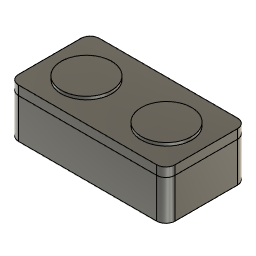
HCSR04-cover (Autodesk Fusion 360 design; units mm, degrees)
Autodesk Fusion 360 part; units mm, degrees
sketch "HCSR04-mock" plane through (0, 0, 0) normal (0, 0, 1) x (1, 0, 0)
  line L0 (0, 0) -> (45.3, 0)
  line L1 (45.3, 0) -> (45.3, 20.5)
  line L2 (45.3, 20.5) -> (0, 20.5)
  line L3 (0, 20.5) -> (0, 0)
  line L4 (22.65, 20.5) -> (22.65, 0) construction
  line L5 (17.525, 3.4) -> (27.775, 3.4)
  line L6 (27.775, 3.4) -> (27.775, 0.4)
  line L7 (27.775, 0.4) -> (17.525, 0.4)
  line L8 (17.525, 0.4) -> (17.525, 3.4)
  line L9 (17.275, 19.75) -> (28.025, 19.75)
  line L10 (28.025, 19.75) -> (28.025, 15.41)
  line L11 (28.025, 15.41) -> (17.275, 15.41)
  line L12 (17.275, 15.41) -> (17.275, 19.75)
  circle A0 centre (9.525, 9.75) radius 8.25
  line L13 (9.525, 9.75) -> (17.775, 9.75) construction
  circle A1 centre (35.775, 9.75) radius 8.25
  line L14 (35.775, 9.75) -> (27.525, 9.75) construction
  line L15 (9.525, 18) -> (9.525, 9.75) construction
  line L16 (35.775, 9.75) -> (35.775, 18)
  line L17 (17.775, 9.75) -> (27.525, 9.75) construction
  line L18 (27.05, 11.795) -> (18.25, 11.795)
  line L19 (18.25, 11.795) -> (18.25, 7.705)
  line L20 (18.25, 7.705) -> (27.05, 7.705)
  line L21 (27.05, 7.705) -> (27.05, 11.795)
  line L22 (27.05, 11.795) -> (18.25, 7.705) construction
  line L23 (18.25, 11.795) -> (27.05, 7.705) construction
  point P0 (22.65, 3.4)
  point P1 (22.65, 19.75)
  point P2 (17.775, 9.75)
  point P3 (27.525, 9.75)
  point P4 (9.525, 18)
  point P5 (35.775, 18)
  point P6 (22.65, 9.75)
  point P7 (22.65, 9.75)
  dimension "d40" = 45.3
  dimension "d41" = 20.5
  dimension "d44" = 10.25
  dimension "d45" = 3
  dimension "d46" = 0.4
  dimension "d47" = 10.75
  dimension "d48" = 4.34
  dimension "d49" = 0.75
  dimension "d50" = 16.5
  dimension "d51" = 16.5
  dimension "d52" = 2.5
  dimension "d53" = 2.5
  dimension "d55" = 9.75
  dimension "d69" = 8.8
  dimension "d70" = 4.09
  constraint horizontal L0
  constraint vertical L1
  constraint horizontal L2
  constraint vertical L3
  constraint coincident L0.start L3.end
  constraint midpoint L2 L4.start
  constraint midpoint L0 L4.end
  constraint horizontal L5
  constraint vertical L6
  constraint horizontal L7
  constraint vertical L8
  constraint midpoint L5 P0
  constraint coincident L4 P0
  constraint horizontal L9
  constraint vertical L10
  constraint horizontal L11
  constraint vertical L12
  constraint midpoint L9 P1
  constraint coincident L4 P1
  constraint coincident A0.centre L13.start
  constraint coincident A0 P2
  constraint horizontal L13
  constraint coincident A1.centre L14.start
  constraint coincident A1 P3
  constraint parallel L11 L14
  constraint coincident P2 L13.end
  constraint coincident P3 L14.end
  constraint coincident A0 P4
  constraint coincident P4 L15.start
  constraint perpendicular L13 L15
  constraint coincident A1 P5
  constraint perpendicular L14 L16
  constraint coincident P5 L16.end
  constraint midpoint L17 P7
  constraint coincident L4 P7
  constraint horizontal L18
  constraint perpendicular L18 L19
  constraint parallel L18 L20
  constraint parallel L19 L21
  constraint coincident L22 P7
  constraint coincident L23 P7
  constraint coincident P7 P6
  measures "d40" distance of L0.start L0.end
  measures "d41" distance of L0.start L2.end
  measures "d44" distance of L5.start L5.end
  measures "d45" distance of L5.start L7.end
  measures "d46" distance of L0 L7
  measures "d47" distance of L9.start L9.end
  measures "d48" distance of L9.start L11.end
  measures "d49" distance of L2 L9
  measures "d50" diameter of A0
  measures "d51" diameter of A1
  measures "d52" distance of L2 P4
  measures "d53" distance of L2 P5
  measures "d55" distance of P2 P3
  measures "d69" distance of L19.end L20.end
  measures "d70" distance of L18.end L19.end
extrude "Extrude9" add sketch "HCSR04-mock" along normal blind 1.2 contours L0 L1 L2 L3 | L5 L6 L7 L8 | L9 L10 L11 L12 | A0 | A1 | L18 L19 L20 L21 makes body 1
extrude "Extrude10" add sketch "HCSR04-mock" along normal blind 12 from surface at 1.2 contours A0 | A1 bodies 1
extrude "Extrude11" add sketch "HCSR04-mock" along normal blind 3.6 from surface at 1.2 contours L9 L10 L11 L12 bodies 1
extrude "Extrude12" add sketch "HCSR04-mock" along normal blind 1.78 from surface at 1.2 contours L5 L6 L7 L8 bodies 1
extrude "Extrude13" add sketch "HCSR04-mock" against normal blind 1.8 contours L5 L6 L7 L8 bodies 1
extrude "Extrude14" add sketch "HCSR04-mock" against normal blind 1.75 contours L18 L19 L20 L21 bodies 1
sketch "Sketch5" plane through (0, 0, 1.2) normal (0, 0, 1) x (-1, 0, 0)
  line L0 (-17.525, -3.4) -> (-27.775, -3.4)
  line L1 (-27.775, -3.4) -> (-27.775, -0.4)
  line L2 (-27.775, -0.4) -> (-17.525, -0.4)
  line L3 (-17.525, -0.4) -> (-17.525, -3.4)
  line L4 (-17.275, -19.75) -> (-28.025, -19.75)
  line L5 (-28.025, -19.75) -> (-28.025, -15.41)
  line L6 (-28.025, -15.41) -> (-17.275, -15.41)
  line L7 (-17.275, -15.41) -> (-17.275, -19.75)
  circle A0 centre (-9.525, -9.75) radius 8.25
  circle A1 centre (-35.775, -9.75) radius 8.25
  line L8 (0, -20.5) -> (0, 0)
  line L9 (0, 0) -> (-45.3, 0)
  line L10 (-45.3, 0) -> (-45.3, -20.5)
  line L11 (-45.3, -20.5) -> (0, -20.5)
  line L12 (3, -23.5) -> (3, 3)
  line L13 (3, 3) -> (-48.3, 3)
  line L14 (-48.3, 3) -> (-48.3, -23.5)
  line L15 (-48.3, -23.5) -> (3, -23.5)
  dimension "d73" = 3
extrude "Extrude15" add sketch "Sketch5" along normal blind 8 and the other way blind 5 separate body contours L0 L1 L2 L3 | L4 L5 L6 L7 | A0 | A1 | L8 L9 L10 L11 | L12 L13 L14 L15 makes body 2
shell "Shell1" thickness 2 removed faces 1 at (14.1, 14.6667, 9.2) on bodies 2
sketch "notch" plane through (0, 21.5, 0) normal (0, -1, 0) x (1, 0, 0)
  line L0 (-1, 9.2) -> (-1, -1.8)
  line L1 (-1, -1.8) -> (46.3, -1.8)
  line L2 (46.3, -1.8) -> (46.3, 9.2)
  line L3 (46.3, 9.2) -> (-1, 9.2)
  line L4 (22.65, 9.2) -> (22.65, 4.2) construction
  line L5 (17.15, 9.2) -> (28.15, 9.2)
  line L6 (28.15, 9.2) -> (28.15, 7.2)
  line L7 (28.15, 7.2) -> (17.15, 7.2)
  line L8 (17.15, 7.2) -> (17.15, 9.2)
  point P0 (22.65, 9.2)
  dimension "d87" = 11
  dimension "d88" = 2
  constraint midpoint L3 P0
  constraint perpendicular L3 L4
  constraint horizontal L5
  constraint vertical L6
  constraint horizontal L7
  constraint vertical L8
  constraint coincident L3 L5.start
  constraint midpoint L5 P0
  constraint coincident L4 P0
  measures "d87" distance of L5.start L5.end
  measures "d88" distance of L5.start L7.end
fillet "Fillet3" radius 3 4 edges at (48.3, -3, 2.7) (48.3, 23.5, 2.7) (-3, -3, 2.7) (-3, 23.5, 2.7) on bodies 2
sketch "top" plane through (0, 0, 9.2) normal (0, 0, 1) x (-1, 0, 0)
  arc A0 (0, -23.5) -> (3, -20.5) centre (0, -20.5) ccw
  line L0 (3, -20.5) -> (3, 0)
  arc A1 (3, 0) -> (0, 3) centre (0, 0) ccw
  line L1 (0, 3) -> (-45.3, 3)
  arc A2 (-45.3, 3) -> (-48.3, 0) centre (-45.3, 0) ccw
  line L2 (-48.3, 0) -> (-48.3, -20.5)
  arc A3 (-48.3, -20.5) -> (-45.3, -23.5) centre (-45.3, -20.5) ccw
  line L3 (-45.3, -23.5) -> (0, -23.5)
  line L4 (-46.3, -21.5) -> (-46.3, 1)
  line L5 (-46.3, 1) -> (1, 1)
  line L6 (1, 1) -> (1, -21.5)
  line L7 (1, -21.5) -> (-46.3, -21.5)
extrude "Extrude16" add sketch "top" along normal blind 3 separate body contours A0 L0 A1 L1 A2 L2 A3 L3 | L4 L5 L6 L7 makes body 3
sketch "top-shell" plane through (0, 0, 9.2) normal (0, 0, -1) x (1, 0, 0)
  line L0 (0, -23.5) -> (45.3, -23.5)
  arc A0 (45.3, -23.5) -> (48.3, -20.5) centre (45.3, -20.5) ccw
  line L1 (48.3, -20.5) -> (48.3, 0)
  arc A1 (48.3, 0) -> (45.3, 3) centre (45.3, 0) ccw
  line L2 (45.3, 3) -> (0, 3)
  arc A2 (0, 3) -> (-3, 0) centre (0, 0) ccw
  line L3 (-3, 0) -> (-3, -20.5)
  arc A3 (-3, -20.5) -> (0, -23.5) centre (0, -20.5) ccw
  line L4 (-0.5, 0) -> (-0.5, -20.5)
  arc A4 (-0.5, -20.5) -> (0, -21) centre (0, -20.5) ccw
  line L5 (0, -21) -> (45.3, -21)
  arc A5 (45.3, -21) -> (45.8, -20.5) centre (45.3, -20.5) ccw
  line L6 (45.8, -20.5) -> (45.8, 0)
  arc A6 (45.8, 0) -> (45.3, 0.5) centre (45.3, 0) ccw
  line L7 (45.3, 0.5) -> (0, 0.5)
  arc A7 (0, 0.5) -> (-0.5, 0) centre (0, 0) ccw
  dimension "d83" = -2.5
extrude "Extrude17" add sketch "top-shell" along normal blind 1.75 contours L4 A4 L5 A5 L6 A6 L7 A7 bodies 3
extrude "Extrude18" add sketch "notch" along normal blind 4 draft -45 contours L3 L5 L6 L7 L8 bodies 2
ref_plane "WorkPlane2" through (22.65, 10.25, 3.7) normal (0, -1, 0) x (1, 0, 0)
mirror "Mirror2" about plane through (22.65, 10.25, 3.7) normal (0, -1, 0) of "Extrude18"
extrude "Extrude20" cut sketch "notch" along normal blind 2.5 draft -40 contours L3 L5 L6 L7 L8 bodies 3
mirror "Mirror3" about plane through (22.65, 10.25, 3.7) normal (0, -1, 0) of "Extrude20"
extrude "Extrude21" cut sketch "HCSR04-mock" along normal blind 2 from surface at -3.8 contours L5 L6 L7 L8 bodies 2
combine "Combine2" operation cut target body 3 tool bodies 1 keep tools
chamfer "Chamfer3" distance 0.2 angle 45 8 edges at (22.65, -0.5, 7.45) (-0.3536, -0.3536, 7.45) (-0.5, 10.25, 7.45) (-0.3536, 20.8536, 7.45) (22.65, 21, 7.45) (45.6536, 20.8536, 7.45) (45.8, 10.25, 7.45) (45.6536, -0.3536, 7.45) on bodies 3
named bodies: "HCSR04-mock", "HCSR04-bottom", "HCSR04-top"
